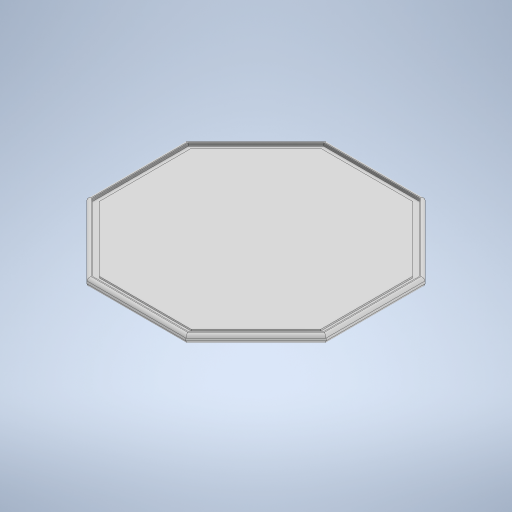
# Autodesk Inventor part: OV-PAM_bottom_2
Saved by Autodesk Inventor 2024 (Build 280153000, 153)
## iProperties
Created: 2023-06-16
Part Number: OV-PAM_bottom_2
Material: 일반
Document SubType Name: Modeling
Designer: jsw
Density: 1 g/cm^3
Appearance: 기본값
Author: jsw
Autodesk Inventor part; units mm, degrees
ref_plane "YZ Plane" through (0, 0, 0) normal (1, 0, 0) x (0, 1, 0)
ref_plane "XZ Plane" through (0, 0, 0) normal (0, 1, 0) x (-1, 0, 0)
ref_plane "XY Plane" through (0, 0, 0) normal (0, 0, 1) x (1, 0, 0)
sketch "스케치3" plane through (0, 0, 0) normal (0, 1, 0) x (-1, 0, 0)
  line L0 (49.0919, -20.3345) -> (20.3345, -49.0919)
  line L1 (20.3345, -49.0919) -> (-20.3345, -49.0919)
  line L2 (-20.3345, -49.0919) -> (-49.0919, -20.3345)
  line L3 (-49.0919, -20.3345) -> (-49.0919, 20.3345)
  line L4 (-49.0919, 20.3345) -> (-20.3345, 49.0919)
  line L5 (-20.3345, 49.0919) -> (20.3345, 49.0919)
  line L6 (20.3345, 49.0919) -> (49.0919, 20.3345)
  line L7 (49.0919, 20.3345) -> (49.0919, -20.3345)
  line L8 (19.0919, -46.0919) -> (-19.0919, -46.0919)
  line L9 (-19.0919, -46.0919) -> (-46.0919, -19.0919)
  line L10 (-46.0919, -19.0919) -> (-46.0919, 19.0919)
  line L11 (-46.0919, 19.0919) -> (-19.0919, 46.0919)
  line L12 (-19.0919, 46.0919) -> (19.0919, 46.0919)
  line L13 (19.0919, 46.0919) -> (46.0919, 19.0919)
  line L14 (46.0919, 19.0919) -> (46.0919, -19.0919)
  line L15 (46.0919, -19.0919) -> (19.0919, -46.0919)
  point P0 (0, 0)
  point P1 (0, 0)
  point P2 (0, 0)
  point P3 (0, 0)
  dimension "d66" = 38.1838
  dimension "d67" = 3
  constraints: 32 end point, 3 coincident, 2 horizontal, 34 other
  measures "d66" distance of L8.start L8.end
  measures "d67" distance between parallel lines of L15 L0
extrude "돌출2" add sketch "스케치3" along normal blind 3.4 contours L0 L1 L2 L3 L4 L5 L6 L7 | L8 L9 L10 L11 L12 L13 L14 L15
sketch "스케치4" plane through (0, 3.4, 0) normal (0, 1, 0) x (1, 0, 0)
  line L0 (18.9262, -45.6919) -> (-18.9262, -45.6919)
  line L1 (-18.9262, -45.6919) -> (-45.6919, -18.9262)
  line L2 (-45.6919, -18.9262) -> (-45.6919, 18.9262)
  line L3 (-45.6919, 18.9262) -> (-18.9262, 45.6919)
  line L4 (-18.9262, 45.6919) -> (18.9262, 45.6919)
  line L5 (18.9262, 45.6919) -> (45.6919, 18.9262)
  line L6 (45.6919, 18.9262) -> (45.6919, -18.9262)
  line L7 (45.6919, -18.9262) -> (18.9262, -45.6919)
  line L8 (-19.6718, 47.4919) -> (19.6718, 47.4919)
  line L9 (19.6718, 47.4919) -> (47.4919, 19.6718)
  line L10 (47.4919, 19.6718) -> (47.4919, -19.6718)
  line L11 (47.4919, -19.6718) -> (19.6718, -47.4919)
  line L12 (19.6718, -47.4919) -> (-19.6718, -47.4919)
  line L13 (-19.6718, -47.4919) -> (-47.4919, -19.6718)
  line L14 (-47.4919, -19.6718) -> (-47.4919, 19.6718)
  line L15 (-47.4919, 19.6718) -> (-19.6718, 47.4919)
  line L16 (-18.8434, 45.4919) -> (18.8434, 45.4919)
  line L17 (18.8434, 45.4919) -> (45.4919, 18.8434)
  line L18 (45.4919, 18.8434) -> (45.4919, -18.8434)
  line L19 (45.4919, -18.8434) -> (18.8434, -45.4919)
  line L20 (18.8434, -45.4919) -> (-18.8434, -45.4919)
  line L21 (-18.8434, -45.4919) -> (-45.4919, -18.8434)
  line L22 (-45.4919, -18.8434) -> (-45.4919, 18.8434)
  line L23 (-45.4919, 18.8434) -> (-18.8434, 45.4919)
  line L24 (-49.0919, 20.3345) -> (-49.0919, -20.3345) projected
  point P0 (0, 0)
  point P1 (0, 0)
  point P2 (0, 0)
  point P3 (0, 0)
  dimension "d68" = 1.8
  dimension "d69" = 0.2
  dimension "d99" = 1.6
  constraints: 48 end point, 3 coincident, 3 horizontal, 51 other
  measures "d68" distance between parallel lines of L3 L15
  measures "d69" distance between parallel lines of L16 L4
  measures "d99" distance between parallel lines of L24 L14
extrude "돌출3" cut sketch "스케치4" against normal blind 1.2 contours L0 L1 L2 L3 L4 L5 L6 L7 | L8 L9 L10 L11 L12 L13 L14 L15 | L16 L17 L18 L19 L20 L21 L22 L23
sketch "스케치9" plane through (0, 0, 0) normal (0, -1, 0) x (1, 0, 0)
  line L0 (7.5, 10) -> (2.5, 10)
  line L1 (2.5, 10) -> (2.5, -10)
  line L2 (2.5, -10) -> (7.5, -10)
  line L3 (7.5, -10) -> (7.5, 10)
  line L4 (7.5, 10) -> (2.5, -10) construction
  line L5 (2.5, 10) -> (7.5, -10) construction
  line L6 (-2.5, 10) -> (-7.5, 10)
  line L7 (-7.5, 10) -> (-7.5, -10)
  line L8 (-7.5, -10) -> (-2.5, -10)
  line L9 (-2.5, 10) -> (-7.5, -10) construction
  line L10 (-7.5, 10) -> (-2.5, -10) construction
  line L11 (-2.5, -10) -> (-2.5, 10)
  point P0 (0, 0)
  point P1 (5, 0)
  point P2 (-5, 0)
  dimension "d42" = 20
  dimension "d43" = 5
  dimension "d44" = 2.5
  dimension "d47" = 10
  constraints: 24 end point, 2 horizontal, 2 midpoint, 2 parallel, 1 collinear, 1 horizontal alignment, 1 perpendicular, 10 other
  measures "d42" distance of L2.end L0.start
  measures "d43" distance of L1.end L2.end
  measures "d44" distance from line of L1 point (0, 0)
  measures "d47" distance of L0.start L6.start
extrude "돌출8" add sketch "스케치9" along normal blind 10
sketch "스케치10" plane through (-7.5, 0, -10) normal (-1, 0, 0) x (0, 0, 1)
  circle A0 centre (15, -5) radius 1.25
  line L0 (19.9591, 0) -> (0.0886, 0)
  line L1 (30.3345, 0) -> (-10.3345, 0) projected
  circle A1 centre (5, -5) radius 1.25
  line L2 (20, 0) -> (20, -10) projected
  point P0 (10, 0)
  dimension "d54" = 2.5
  dimension "d57" = 10
  dimension "d62" = 5
  dimension "d63" = 5
  constraints: 2 centre point, 2 end point, 1 horizontal, 1 point on line, 2 other
  measures "d54" diameter of A0
  measures "d57" distance of A0.centre A1.centre
  measures "d62" distance from line of L0 A0.centre
  measures "d63" distance from line of L2 A0.centre
extrude "돌출9" cut sketch "스케치10" against normal blind 20
sketch "스케치11" plane through (0, 2.2, 0) normal (0, 1, 0) x (1, 0, 0)
  line L0 (-18.8434, 45.4919) -> (18.8434, 45.4919)
  line L1 (18.8434, 45.4919) -> (45.4919, 18.8434)
  line L2 (45.4919, 18.8434) -> (45.4919, -18.8434)
  line L3 (45.4919, -18.8434) -> (18.8434, -45.4919)
  line L4 (18.8434, -45.4919) -> (-18.8434, -45.4919)
  line L5 (-18.8434, -45.4919) -> (-45.4919, -18.8434)
  line L6 (-45.4919, -18.8434) -> (-45.4919, 18.8434)
  line L7 (-45.4919, 18.8434) -> (-18.8434, 45.4919)
  line L8 (-19.6718, 47.4919) -> (19.6718, 47.4919) projected
  line L9 (-17.6007, 42.4919) -> (17.6007, 42.4919)
  line L10 (17.6007, 42.4919) -> (42.4919, 17.6007)
  line L11 (42.4919, 17.6007) -> (42.4919, -17.6007)
  line L12 (42.4919, -17.6007) -> (17.6007, -42.4919)
  line L13 (17.6007, -42.4919) -> (-17.6007, -42.4919)
  line L14 (-17.6007, -42.4919) -> (-42.4919, -17.6007)
  line L15 (-42.4919, -17.6007) -> (-42.4919, 17.6007)
  line L16 (-42.4919, 17.6007) -> (-17.6007, 42.4919)
  point P0 (0, 0)
  point P1 (0, 0)
  point P2 (0, 0)
  dimension "d70" = 2
  dimension "d71" = 3
  constraints: 32 end point, 2 coincident, 2 horizontal, 34 other
  measures "d70" distance between parallel lines of L8 L0
  measures "d71" distance between parallel lines of L9 L0
extrude "돌출10" add sketch "스케치11" along normal blind 0.6 contours L0 L1 L2 L3 L4 L5 L6 L7 | L9 L10 L11 L12 L13 L14 L15 L16
fillet "모깎기1" radius 1.2 16 edges at (-34.7132, 3.4, 34.7132) (0, 3.4, 49.0919) (34.7132, 3.4, 34.7132) (49.0919, 3.4, 0) (34.7132, 3.4, -34.7132) (0, 3.4, -49.0919) (-34.7132, 3.4, -34.7132) (-49.0919, 3.4, 0) (-34.7132, 0, 34.7132) (0, 0, 49.0919) (34.7132, 0, 34.7132) (49.0919, 0, 0) (34.7132, 0, -34.7132) (0, 0, -49.0919) (-34.7132, 0, -34.7132) (-49.0919, 0, 0)
